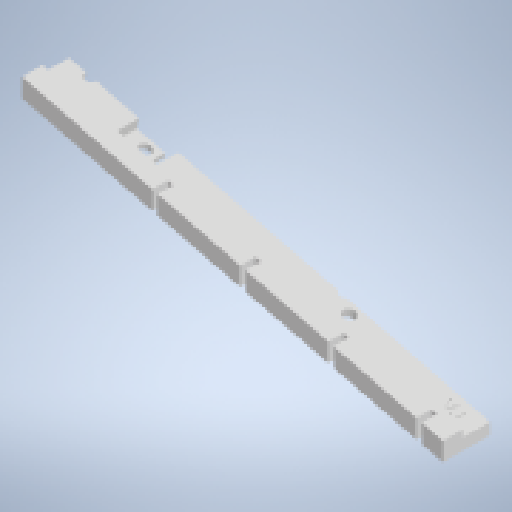
# Autodesk Inventor part: A1200net Left mount
Saved by Autodesk Inventor 2025 (Build 290162000, 162)
## iProperties
Created: 2024-07-17
Part Number: A1200net Left mount
Material: Generic
Document SubType Name: Modeling
Designer: adam
Density: 1 g/cm^3
Appearance: Default
Author: adam
Autodesk Inventor part; units mm, degrees
ref_plane "YZ Plane" through (0, 0, 0) normal (1, 0, 0) x (0, 1, 0)
ref_plane "XZ Plane" through (0, 0, 0) normal (0, 1, 0) x (-1, 0, 0)
ref_plane "XY Plane" through (0, 0, 0) normal (0, 0, 1) x (1, 0, 0)
sketch "Sketch1" plane through (0, 0, 0) normal (0, 0, 1) x (1, 0, 0)
  line L0 (0, 0) -> (-125.1681, 31.2079)
  line L1 (0, 0) -> (-48.3113, 0) construction
  line L2 (0, 0) -> (0, 5.5)
  line L3 (-125.1681, 31.2079) -> (-125.1681, 36.7079)
  line L4 (-125.1681, 36.7079) -> (0, 5.5)
  dimension "d0" = 14
  dimension "d1" = 129
  dimension "d2" = 5.5
  dimension "d3" = 5.5
  constraints: 10 end point, 1 horizontal, 1 perpendicular, 1 vertical
  measures "d0" angle of L1 L0
  measures "d1" distance of L0.start L0.end
  measures "d2" distance of L0.start L2.end
  measures "d3" distance of L0.end L3.end
extrude "Side rail" add sketch "Sketch1" against normal blind 6
sketch "Sketch2" plane through (0, 0, 0) normal (0, 0, 1) x (1, 0, 0)
  line L0 (-125.1681, 36.7079) -> (0, 5.5) projected
  line L1 (-6.3069, 7.0725) -> (-6.3069, 1.5725)
  line L2 (0, 0) -> (-125.1681, 31.2079) projected
  line L3 (0, 5.5) -> (-125.1681, 36.7079) construction
  line L4 (-125.1681, 36.7079) -> (-125.1681, 31.2079) construction
  line L5 (-125.1681, 31.2079) -> (0, 0) construction
  line L6 (0, 0) -> (0, 5.5) construction
  line L7 (-6.3069, 7.0725) -> (-7.8569, 7.459)
  line L8 (-7.8569, 7.459) -> (-7.8569, 1.959)
  line L9 (-7.8569, 1.959) -> (-6.3069, 1.5725)
  line L10 (-32.5049, 13.6044) -> (-32.5049, 8.1044)
  line L11 (-32.5049, 8.1044) -> (-34.0549, 8.4908)
  line L12 (-34.0549, 8.4908) -> (-34.0549, 13.9908)
  line L13 (-34.0549, 13.9908) -> (-32.5049, 13.6044)
  line L14 (-58.7029, 20.1363) -> (-58.7029, 14.6363)
  line L15 (-58.7029, 14.6363) -> (-60.2529, 15.0227)
  line L16 (-60.2529, 15.0227) -> (-60.2529, 20.5227)
  line L17 (-60.2529, 20.5227) -> (-58.7029, 20.1363)
  line L18 (-58.7029, 20.1363) -> (-60.2529, 20.1363) construction
  line L19 (-32.5049, 13.6044) -> (-34.0549, 13.6044) construction
  line L20 (-6.3069, 7.0725) -> (-7.8569, 7.0725) construction
  line L21 (-84.9009, 26.6682) -> (-84.9009, 21.1682)
  line L22 (-84.9009, 21.1682) -> (-86.4509, 21.5546)
  line L23 (-86.4509, 21.5546) -> (-86.4509, 27.0546)
  line L24 (-86.4509, 27.0546) -> (-84.9009, 26.6682)
  line L25 (-84.9009, 26.6682) -> (-86.4509, 26.6682) construction
  line L26 (0, 5.5) -> (-125.1681, 36.7079) projected
  line L27 (-125.1681, 31.2079) -> (0, 0) projected
  point P0 (-7.8569, 1.959)
  point P1 (-34.0549, 8.4908)
  point P2 (-32.5049, 8.1044)
  point P3 (-32.5049, 13.6044)
  point P4 (-60.2529, 20.5227)
  point P5 (-60.2529, 15.0227)
  point P6 (-58.7029, 20.1363)
  dimension "d6" = 1.55
  dimension "d7" = 6.5
  dimension "d8" = 33.5
  dimension "d9" = 60.5
  dimension "d15" = 87.5
  constraints: 40 end point, 16 point on line, 8 parallel, 5 collinear, 4 vertical, 3 perpendicular, 2 other
  measures "d6" distance of L1.start L20.end
  measures "d7" distance of L2.start L1.end
  measures "d8" distance of L2.start L10.end
  measures "d9" distance of L2.start L14.end
  measures "d15" distance of L2.start L21.end
extrude "Side rail cuts" cut sketch "Sketch2" against normal blind 4.5 contours L0 L21 L2 L23 | L0 L14 L2 L16 | L0 L10 L2 L12 | L0 L1 L2 L8
sketch "Sketch3" plane through (0, 0, -6) normal (0, 0, -1) x (-1, 0, 0)
  line L0 (0, 0) -> (125.1681, 31.2079) projected
  line L1 (0, 0) -> (0, 5.5) projected
  line L2 (0, 3.4388) -> (125.1681, 34.6467)
  line L3 (125.1681, 36.7079) -> (125.1681, 31.2079) projected
  line L4 (0, 3.4388) -> (0, 0)
  line L5 (125.1681, 34.6467) -> (125.1681, 31.2079)
  line L6 (125.1681, 36.7079) -> (0, 5.5) projected
  dimension "d12" = 2
  constraints: 6 end point, 2 collinear, 2 point on line
  measures "d12" distance between parallel lines of L2 L6
extrude "Keyboard support" add sketch "Sketch3" along normal blind 8 contours L1 L2 L3 L0
sketch "Sketch4" plane through (0, 3.4388, -6) normal (0.2419219, 0.9702957, 0) x (0.9702957, -0.2419219, 0)
  line L0 (-129, 0) -> (-129, 8) construction
  line L1 (-129, 5) -> (0, 5) construction
  line L2 (0, 0) -> (0, 8) construction
  line L3 (0, 0) -> (-129, 0) construction
  circle A0 centre (-40, 5) radius 1.75
  line L4 (0.8319, 8) -> (-128.1681, 8) projected
  line L5 (-95.5, 8) -> (-95.5, 0)
  line L6 (-107.5, 0) -> (-107.5, 8)
  line L7 (-107.5, 8) -> (-95.5, 8)
  line L8 (-107.5, 0) -> (-95.5, 0)
  point P0 (0.8319, -6)
  dimension "d16" = 5
  dimension "d17" = 40
  dimension "d18" = 95.5
  dimension "d19" = 12
  dimension "d20" = 3.5
  constraints: 10 end point, 7 point on line, 2 collinear, 2 perpendicular, 1 centre point, 1 horizontal
  measures "d16" distance between parallel lines of L1 L3
  measures "d17" distance from line of L2 A0.centre
  measures "d18" distance between parallel lines of L2 L5
  measures "d19" distance between parallel lines of L5 L6
  measures "d20" diameter of A0
extrude "Mount hole and brace clearance" cut sketch "Sketch4" against normal up to surface (3.3366 mm away)
sketch "Sketch5" plane through (0, 0, -6) normal (0, 0, -1) x (-1, 0, 0)
  line L0 (125.1681, 34.6467) -> (104.3068, 29.4454) construction
  line L1 (104.3068, 29.4454) -> (92.6269, 26.5333) construction
  line L2 (104.3068, 29.4454) -> (105.114, 26.2079) projected
  line L3 (105.0326, 26.5345) -> (96.494, 24.4056)
  line L4 (96.494, 24.4056) -> (96.8568, 22.9501)
  line L5 (96.8568, 22.9501) -> (111.4113, 26.579)
  line L6 (111.4113, 26.579) -> (111.0484, 28.0344)
  line L7 (111.0484, 28.0344) -> (105.0326, 26.5345)
  line L8 (93.4704, 23.3048) -> (92.6632, 26.5423) projected
  point P0 (0, 0)
  dimension "d23" = 3
  dimension "d24" = 1.5
  dimension "d25" = 3.2
  dimension "d26" = 15
  constraints: 12 end point, 4 perpendicular, 1 collinear, 1 point on line
  measures "d23" distance between parallel lines of L3 L1
  measures "d24" distance between parallel lines of L5 L3
  measures "d25" distance between parallel lines of L4 L8
  measures "d26" distance between parallel lines of L6 L4
extrude "Brace support" add sketch "Sketch5" along normal blind 8 and the other way blind 3.3
sketch "Sketch6" plane through (-96.494, 24.4056, -6) normal (0.2419219, 0.9702957, 0) x (0.9702957, -0.2419219, 0)
  circle A0 centre (-3.3, 5) radius 1.75
  circle A1 centre (58.7, 5) radius 1.75 construction
  line L0 (-30.7987, 0) -> (98.2013, 0) construction
  line L1 (98.7, 0) -> (98.7, 8) construction
  point P0 (99.5319, -6)
  dimension "d31" = 5
  dimension "d32" = 102
  constraints: 1 centre point, 1 equal radius
  measures "d31" distance from line of A0.centre L0
  measures "d32" distance from line of L1 A0.centre
extrude "Extrusion6" cut sketch "Sketch6" against normal up to surface (1.5 mm away)
sketch "Sketch8" plane through (0, 0, -14) normal (-0.2419219, -0.9702957, 0) x (0.9702957, -0.2419219, 0)
  circle A0 centre (-40.8319, 3) radius 1.75 projected
  arc A1 (-37.0819, 3) -> (-44.5819, 3) centre (-40.8319, 3) ccw
  line L0 (0, 0) -> (-96.3319, 0) projected
  line L1 (-37.0819, 3) -> (-37.0819, 0)
  line L2 (-44.5819, 3) -> (-44.5819, 0)
  point P0 (0, 14)
  dimension "d40" = 7.5
  constraints: 4 end point, 2 perpendicular, 2 point on circle, 2 point on line, 2 tangent, 1 centre point, 1 coincident
  measures "d40" diameter of A1
extrude "Extrusion8" cut sketch "Sketch8" against normal blind 1
sketch "Sketch9" plane through (-6.3069, 1.5725, -4.5) normal (-0.2419219, -0.9702957, 0) x (0.9702957, -0.2419219, 0)
  circle A0 centre (-116.4884, -9.265) radius 0.725 construction
  arc A1 (-114.9884, -9.265) -> (-117.9884, -9.265) centre (-116.4884, -9.265) ccw
  line L0 (-117.9884, -9.265) -> (-117.9884, -9.5)
  line L1 (-123.3319, -9.5) -> (-101.8319, -9.5) construction
  line L2 (-114.9884, -9.265) -> (-114.9884, -9.5)
  line L3 (-114.9884, -9.5) -> (-117.9884, -9.5)
  circle A2 centre (-39.3839, -10.2145) radius 0.725 construction
  arc A3 (-38.065, -9.5) -> (-40.7028, -9.5) centre (-39.3839, -10.2145) ccw
  line L4 (-38.0819, -9.5) -> (-89.8319, -9.5) construction
  line L5 (-40.7028, -9.5) -> (-37.9571, -9.5) construction
  line L6 (-89.8319, -9.5) -> (5.6681, -9.5) projected
  line L7 (-38.065, -9.5) -> (-40.7028, -9.5)
  point P0 (6.5, 4.5)
  dimension "d46" = 3
  dimension "d47" = 3
  constraints: 10 end point, 4 point on circle, 4 point on line, 3 collinear, 2 centre point, 2 coincident, 2 tangent, 1 perpendicular, 1 vertical
  measures "d46" diameter of A1
  measures "d47" diameter of A3
extrude "Extrusion9" cut sketch "Sketch9" against normal up to surface (3.3366 mm away)
sketch "Sketch10" plane through (0, 5.5, 0) normal (0.2419219, 0.9702957, 0) x (0.9702957, -0.2419219, 0)
  line L0 (-50.1535, 9.9846) -> (-44.0945, 9.9846) construction
  line L1 (-44.0945, 9.9846) -> (-44.0945, 6.9267) construction
  line L2 (-44.0945, 6.9267) -> (-50.1535, 6.9267) construction
  line L3 (-50.1535, 6.9267) -> (-50.1535, 9.9846) construction
  line L4 (-47.8881, 9.9846) -> (-47.4528, 9.9846)
  line L5 (-47.4528, 9.9846) -> (-48.7411, 6.9219)
  line L6 (-48.7411, 6.9219) -> (-48.8423, 6.9219)
  line L7 (-48.8423, 6.9219) -> (-50.1535, 9.9846)
  line L8 (-50.1535, 9.9846) -> (-49.713, 9.9846)
  line L9 (-49.713, 9.9846) -> (-48.7968, 7.8433)
  line L10 (-48.7968, 7.8433) -> (-47.8881, 9.9846)
  spline S0 degree 2 poles (-46.9668, 7.4206) (-46.8554, 7.4206) (-46.6985, 7.2687) (-46.6985, 7.1573) knots 0 0 0 1 2 2 2
  spline S1 degree 2 poles (-46.6985, 7.1573) (-46.6985, 7.0485) (-46.8529, 6.8991) (-46.9668, 6.8991) knots 0 0 0 1 2 2 2
  spline S2 degree 2 poles (-46.9668, 6.8991) (-47.0782, 6.8991) (-47.23, 7.0485) (-47.23, 7.1573) knots 0 0 0 1 2 2 2
  spline S3 degree 2 poles (-47.23, 7.1573) (-47.23, 7.2687) (-47.0782, 7.4206) (-46.9668, 7.4206) knots 0 0 0 1 2 2 2
  line L11 (-45.5696, 9.9846) -> (-45.1343, 9.9846)
  line L12 (-45.1343, 9.9846) -> (-45.1343, 6.9346)
  line L13 (-45.1343, 6.9346) -> (-45.5696, 6.9346)
  line L14 (-45.5696, 6.9346) -> (-45.5696, 9.9846)
  point P0 (1.3306, 0)
  constraints: 2 other
extrude "Extrusion10" cut sketch "Sketch10" against normal blind 0.5
sketch "Sketch11" plane through (0, 3.4388, -6) normal (0.2419219, 0.9702957, 0) x (0.9702957, -0.2419219, 0)
  line L0 (-70.0252, 6.7194) -> (-59.9721, 6.7194) construction
  line L1 (-59.9721, 6.7194) -> (-59.9721, 1.5) construction
  line L2 (-59.9721, 1.5) -> (-70.0252, 1.5) construction
  line L3 (-70.0252, 1.5) -> (-70.0252, 6.7194) construction
  line L4 (-129.4987, 0) -> (-0.4987, 0) construction
  line L5 (-64.9987, 0) -> (-64.9987, 8.0462) construction
  line L6 (-64.7555, 6.7194) -> (-67.0709, 1.653)
  line L7 (-67.0709, 1.653) -> (-67.6103, 1.653)
  line L8 (-67.6103, 1.653) -> (-70.0252, 6.7194)
  line L9 (-70.0252, 6.7194) -> (-68.6684, 6.7194)
  line L10 (-68.6684, 6.7194) -> (-67.3489, 3.8646)
  line L11 (-67.3489, 3.8646) -> (-66.0957, 6.7194)
  line L12 (-66.0957, 6.7194) -> (-64.7555, 6.7194)
  spline S0 degree 2 poles (-64.4028, 2.292) (-64.4028, 2.5493) (-64.0252, 2.9269) (-63.7638, 2.9269) knots 0 0 0 1 2 2 2
  spline S1 degree 2 poles (-63.7638, 2.9269) (-63.5024, 2.9269) (-63.1248, 2.5493) (-63.1248, 2.292) knots 0 0 0 1 2 2 2
  spline S2 degree 2 poles (-63.1248, 2.292) (-63.1248, 2.0264) (-63.5024, 1.653) (-63.7638, 1.653) knots 0 0 0 1 2 2 2
  spline S3 degree 2 poles (-63.7638, 1.653) (-64.0252, 1.653) (-64.4028, 2.0264) (-64.4028, 2.292) knots 0 0 0 1 2 2 2
  line L13 (-60.2119, 6.7194) -> (-60.2119, 1.7194)
  line L14 (-60.2119, 1.7194) -> (-61.3157, 1.7194)
  line L15 (-61.3157, 1.7194) -> (-61.3157, 6.7194)
  line L16 (-61.3157, 6.7194) -> (-60.2119, 6.7194)
  point P0 (0.8319, -6)
  point P1 (-64.9987, 1.5)
  dimension "d54" = 1.5
  constraints: 2 end point, 2 midpoint, 1 perpendicular, 1 point on line, 2 other
  measures "d54" distance between parallel lines of L4 L2
extrude "Extrusion11" cut sketch "Sketch11" against normal blind 0.5
equation "\"d47\" = d46"
body "Solid1"
